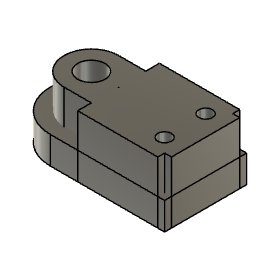
3D Plancha 10 (Autodesk Fusion 360 design; units mm, degrees)
Autodesk Fusion 360 part; units mm, degrees
sketch "Boceto1" plane through (0, 0, 0) normal (0, 0, 1) x (1, 0, 0)
  line L0 (-53.605, 50) -> (30, 50)
  line L1 (30, 50) -> (30, -10)
  line L2 (30, -10) -> (-53.605, -10)
  circle A0 centre (-53.605, 20) radius 10
  line L3 (25, 50) -> (30, 50)
  line L4 (30, 50) -> (30, 45)
  line L5 (30, 45) -> (25, 45)
  line L6 (25, 45) -> (25, 50)
  line L7 (30, -10) -> (25, -10)
  line L8 (25, -10) -> (25, -5)
  line L9 (25, -5) -> (30, -5)
  line L10 (30, -5) -> (30, -10)
  circle A1 centre (15, 5) radius 5
  circle A2 centre (15, 35) radius 5
  arc A3 (-53.605, 50) -> (-53.605, -10) centre (-53.605, 20) ccw
  line L11 (-33.7768, 40) -> (-33.8631, 50)
  arc A4 (-53.605, 40) -> (-53.605, 0) centre (-53.605, 20) ccw
  arc A5 (-33.6057, 19.8275) -> (-33.6057, 20.1725) centre (-53.605, 20) ccw
  line L12 (-53.605, 40) -> (-33.7768, 40)
  line L13 (-53.605, 0) -> (-33.6057, 0)
  line L14 (-33.6057, 22.9183) -> (-33.6057, 19.8275)
  line L15 (-33.6057, 0) -> (-33.6057, -10)
  constraint horizontal L0
  constraint vertical L1
  constraint horizontal L2
  constraint horizontal L3
  constraint vertical L4
  constraint horizontal L5
  constraint vertical L6
  constraint coincident L0 L3.start
  constraint horizontal L7
  constraint vertical L8
  constraint horizontal L9
  constraint vertical L10
  constraint concentric A0 A4
  constraint concentric A0 A3
  constraint coincident L0 L11.end
  constraint tangent L11 A4
  constraint coincident L2 L15.end
  constraint perpendicular L2 L14
  constraint concentric A4 A5
  constraint tangent A4 L12
  constraint coincident L13.end L14
  constraint tangent A4 L13
  constraint collinear L14 L15
extrude "Extruir1" add sketch "Boceto1" along normal blind 20 contours L0 L2 A3 L11 A4 L12 L13 L15 | L0 L1 L2 L5 L6 L8 L9 L11 A4 L12 L13 L15 | L0 L1 L3 L4 L5 L6 | L1 L2 L7 L8 L9 L10 | A0 | A1 | A2 makes body 1
extrude "Extruir2" add sketch "Boceto1" along normal blind 45 separate body contours L0 L1 L2 L5 L6 L8 L9 L11 A4 L12 L13 L15 makes body 2
